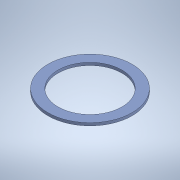
# Autodesk Inventor part: Pump-Motor-CW-Rotation:Gasket 103
Saved by Autodesk Inventor 2022.2 (Build 262287010, 287A)
## iProperties
Created: 2025-06-16
Material: Rubber
Document SubType Name: Modeling
Density: 0.93 g/cm^3
Appearance: Rubber - Blue
Designer: cw
Author: cw
Autodesk Inventor part; units mm, degrees
ref_plane "YZ Plane" through (0, 0, 0) normal (1, 0, 0) x (0, 1, 0)
ref_plane "XZ Plane" through (0, 0, 0) normal (0, 1, 0) x (-1, 0, 0)
ref_plane "XY Plane" through (0, 0, 0) normal (0, 0, 1) x (1, 0, 0)
sketch "Sketch1" plane through (0, 0, 0) normal (0, 0, 1) x (1, 0, 0)
  circle A0 centre (0, 0) radius 23
  circle A1 centre (0, 0) radius 17.5
  dimension "d0" = 46
  dimension "d1" = 35
  constraints: 2 centre point, 2 coincident
  measures "d0" diameter of A0
  measures "d1" diameter of A1
extrude "Extrusion1" add sketch "Sketch1" along normal blind 1.5
body "Solid1"
